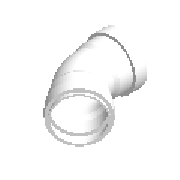
# Autodesk Inventor part: ISO 3633 45 Deg Bend with Only Sockets for Elastomeric Sealing Ring Joints DN160
Saved by Autodesk Inventor 2023.1 (Build 271208000, 208)
## iProperties
Created: 2022-02-04
Part Number: ISO 3633 45 Deg Bend with Only Sockets for Elastomeric Sealing Ring Joints DN160
Material: PVC, Unplasticized
Description: Unplasticized poly(vinylchloride) (PVC-U) - Bend with Only Sockets for Elastomeric Sealing Ring Joints
Document SubType Name: Modeling
Standard: ISO 3633
Designer: user
Standard Revision: Second edition 2002-09-01
Standards Organization: ISO
Language: en-US
Size Designation: DN160
Categories: <MemberInstance><Categories><Category DisplayName="Tube &amp; Pipe" InternalName="4347fa0f-2144-441d-94cd-e3e15c92b736" Mnemonic="TUBEANDPIPE"><CategoryParameter DisplayName="Number of Connections" InternalName="04e9c83a-9e20-4a98-a7e1-e8abe87a2846" Mnemonic="NUM_CONNECTIONS"/><CategoryParameter DisplayName="Angles" InternalName="0e0e4fa4-3bd3-4656-a22e-4e07c8c476f8" Mnemonic="ANGLES"><CategoryParameter DisplayName="Angle" InternalName="9188ad83-1b16-48b4-8b0a-76ce729dafa7" Mnemonic="ANGLE"/></CategoryParameter><CategoryParameter DisplayName="SKey" InternalName="3da84699-049a-4bc2-a65a-6696b77c242f" Mnemonic="SKEY"/><CategoryParameter DisplayName="ISOGEN Description" InternalName="7aa3ba45-b821-4467-8584-f9e6f15f2a7d" Mnemonic="ISOGENDESC"/><CategoryParameter DisplayName="ITEM-CODE" InternalName="99cc3b15-24d9-4d38-aac7-792cfbc57acf" Mnemonic="ITEMCODE"/><CategoryParameter DisplayName="NameOfComponent" InternalName="9c74ad13-48a1-45fe-b0f7-5447561f444a" Mnemonic="NAMEOFCOMPONENT"/><CategoryParameter DisplayName="InLineGroups" InternalName="d60be647-bc43-4c18-a13f-9fe4115f8e64" Mnemonic="INLINEGROUPS"/><Category DisplayName="Fittings" InternalName="ed6b26c4-72b8-4f31-9b63-f85ae8f932e4" Mnemonic="FITTINGS"><CategoryParameter DisplayName="Connections" InternalName="dbd721e8-e885-4eea-9011-b5acfd9f61de" Mnemonic="FIT_CONNECTIONS"><CategoryParameter DisplayName="Min Mating Pipe Size" InternalName="11f51b32-3e37-4310-abf7-f1318a1fd129" Mnemonic="MNMPS"/><CategoryParameter DisplayName="MaxEngagement" InternalName="34fdf028-8797-436e-ba07-ca3dee15bd9b" Mnemonic="MAXENGAGEMENT"/><CategoryParameter DisplayName="NominalSize" InternalName="3f94edc7-e459-48db-8f02-8eebf8cffccd" Mnemonic="NS"/><CategoryParameter DisplayName="DisplayName" InternalName="50f521dd-e050-43f7-9895-6b30ea7ed42e" Mnemonic="DISPLAYNAME"/><CategoryParameter DisplayName="Cut Mating Pipe" InternalName="53a63a6e-53d8-4ca9-8880-037731d1cceb" Mnemonic="CMP"/><CategoryParameter DisplayName="Gender Neutral" InternalName="628bd5f1-acad-44e2-9d91-af996ab74fc2" Mnemonic="NEUTRAL"/><CategoryParameter DisplayName="MinEngagement [% of MaxEngagement]" InternalName="7ec1bde5-73f0-45b1-98d8-365a6c67f8ad" Mnemonic="MINENGAGEMENT"/><CategoryParameter DisplayName="Fixed" InternalName="9142902a-6a8a-446d-9eb8-4b7ce7d245ef" Mnemonic="FIXED"/><CategoryParameter DisplayName="Female" InternalName="b366bcb5-a500-4bad-84bb-22f956216d69" Mnemonic="FEMALE"/><CategoryParameter DisplayName="FlipDirection" InternalName="d55dedc0-f14a-4283-86b4-a4eeb253c8aa" Mnemonic="FLIPDIRECTION"/><CategoryParameter DisplayName="ScheduleNumber" InternalName="d6161c62-eb59-4495-a086-874847c10866" Mnemonic="SN"/><CategoryParameter DisplayName="EndTreatment" InternalName="d7f11516-3374-45ca-b1c7-4b2d63244ae2" Mnemonic="ENDTREATMENT"/><CategoryParameter DisplayName="Max Mating Pipe Size" InternalName="e73ef66b-c04b-45ac-9b32-f712653e25ee" Mnemonic="MXMPS"/></CategoryParameter><CategoryParameter DisplayName="Connections" InternalName="dbd721e8-e885-4eea-9011-b5acfd9f61de" Mnemonic="FIT_CONNECTIONS"><CategoryParameter DisplayName="Min Mating Pipe Size" InternalName="11f51b32-3e37-4310-abf7-f1318a1fd129" Mnemonic="MNMPS"/><CategoryParameter DisplayName="MaxEngagement" InternalName="34fdf028-8797-436e-ba07-ca3dee15bd9b" Mnemonic="MAXENGAGEMENT"/><CategoryParameter DisplayName="NominalSize" InternalName="3f94edc7-e459-48db-8f02-8eebf8cffccd" Mnemonic="NS"/><CategoryParameter DisplayName="DisplayName" InternalName="50f521dd-e050-43f7-9895-6b30ea7ed42e" Mnemonic="DISPLAYNAME"/><CategoryParameter DisplayName="Cut Mating Pipe" InternalName="53a63a6e-53d8-4ca9-8880-037731d1cceb" Mnemonic="CMP"/><CategoryParameter DisplayName="Gender Neutral" InternalName="628bd5f1-acad-44e2-9d91-af996ab74fc2" Mnemonic="NEUTRAL"/><CategoryParameter DisplayName="MinEngagement [% of MaxEngagement]" InternalName="7ec1bde5-73f0-45b1-98d8-365a6c67f8ad" Mnemonic="MINENGAGEMENT"/><CategoryParameter DisplayName="Fixed" InternalName="9142902a-6a8a-446d-9eb8-4b7ce7d245ef" Mnemonic="FIXED"/><CategoryParameter DisplayName="Female" InternalName="b366bcb5-a500-4bad-84bb-22f956216d69" Mnemonic="FEMALE"/><CategoryParameter DisplayName="FlipDirection" InternalName="d55dedc0-f14a-4283-86b4-a4eeb253c8aa" Mnemonic="FLIPDIRECTION"/><CategoryParameter DisplayName="ScheduleNumber" InternalName="d6161c62-eb59-4495-a086-874847c10866" Mnemonic="SN"/><CategoryParameter DisplayName="EndTreatment" InternalName="d7f11516-3374-45ca-b1c7-4b2d63244ae2" Mnemonic="ENDTREATMENT"/><CategoryParameter DisplayName="Max Mating Pipe Size" InternalName="e73ef66b-c04b-45ac-9b32-f712653e25ee" Mnemonic="MXMPS"/></CategoryParameter><Category DisplayName="Elbows" InternalName="d634b27c-b107-44eb-a6d6-89e046173c17" Mnemonic="Elbow"/></Category></Category><Category DisplayName="DataType" InternalName="23b78d0f-2648-40c6-8793-ca6db495c9e8" Mnemonic="DATATYPE"><CategoryParameter DisplayName="DisplayName" InternalName="05415f3d-3907-474b-a020-eb9d644f4cf3" Mnemonic="DISPLAYNAME"/><CategoryParameter DisplayName="Standard" InternalName="0c0a119c-1e12-4c84-803f-101930972f5e" Mnemonic="STANDARD"/><CategoryParameter DisplayName="Description" InternalName="13903e3d-64b1-4950-80da-f627842ea37f" Mnemonic="DESCRIPTION"/><CategoryParameter DisplayName="Designation" InternalName="2675968c-4ce5-49e0-a4f5-552d29089031" Mnemonic="DESIGNATION"/><CategoryParameter DisplayName="Default Row" InternalName="2af9ec52-faaa-4026-b378-f9fa4afca842" Mnemonic="DEFAULTROW"/><CategoryParameter DisplayName="Folder Name" InternalName="3f06958e-8713-4116-9be7-ed6184ecc97b" Mnemonic="FOLDERNAME"/><CategoryParameter DisplayName="Revision Guid" InternalName="45a75005-10b1-4dfc-8d6d-dfe629f0b93c" Mnemonic="REVISIONGUID"/><CategoryParameter DisplayName="FileName" InternalName="8b46a4cc-9585-4fed-90c3-899f57e09a73" Mnemonic="FILENAME"/><CategoryParameter DisplayName="StdsOrg" InternalName="8f5914e1-4693-403f-8ab5-d37768198c9d" Mnemonic="STDSORG"/><CategoryParameter DisplayName="Family Version" InternalName="914462f6-6e19-4b14-ba84-155b9680b1d0" Mnemonic="FAMILYREVISION"/><CategoryParameter DisplayName="Standard Revision" InternalName="91d5a463-65c2-4fde-b823-3b7fea5e8e17" Mnemonic="STANDARDREVISION"/><CategoryParameter DisplayName="Member Revision" InternalName="a65d44b9-392f-4f4f-857b-e4b3d54996fe" Mnemonic="MEMBERREVISION"/><CategoryParameter DisplayName="ClipFormat" InternalName="bc51e27b-3422-4e78-93ef-cec197ddf230" Mnemonic="CLIPFORMAT"/><CategoryParameter DisplayName="Manufacturer" InternalName="cd6c7a72-a28a-4e50-99a9-2c7f4e13e5ad" Mnemonic="MANUFACTURER"/><CategoryParameter DisplayName="InternalName" InternalName="cf1d0246-76d9-4b4a-8305-fa0409afb5c1" Mnemonic="INTERNALNAME"/><CategoryParameter DisplayName="IsMetric" InternalName="e2385c5b-1ea4-4823-96a8-8de651266ec3" Mnemonic="ISMETRIC"/><Category DisplayName="Part" InternalName="c0e0b642-3bcb-4cc8-9e80-f96d35c4afa4" Mnemonic="PART"><CategoryParameter DisplayName="Part Number" InternalName="016b6077-bfbe-49bd-92c9-d8d59c39c941" Mnemonic="PARTNUMBER"/><CategoryParameter DisplayName="Stock Number" InternalName="4dba7c1c-e26c-444e-836c-b08b433409a8" Mnemonic="STOCKNUMBER"/><CategoryParameter DisplayName="Material Key" InternalName="5c9a8adb-dd2b-4535-b97f-0a94a95fe41f" Mnemonic="MATERIALKEY"/><CategoryParameter DisplayName="Material" InternalName="818a152a-d3c3-49ca-80ee-df7d91421b8e" Mnemonic="MATERIAL"/></Category></Category><Category DisplayName="LegacyMap" InternalName="dfeab48a-acc2-4514-a11c-1b8dc28c3d5f" Mnemonic="LEGACYMAP"><CategoryParameter DisplayName="CatalogID" InternalName="0da51c36-8fd3-4028-86cc-0c9c9e96136a" Mnemonic="CATALOGID"/><CategoryParameter DisplayName="FamilyID" InternalName="1c0b589c-8bbe-4e1e-80cf-07c0de42ac2a" Mnemonic="FAMILYID"/><CategoryParameter DisplayName="MemberID" InternalName="a368ea03-db8a-4d6e-962b-2aa46306b8f5" Mnemonic="MEMBERID"/></Category></Categories><FamilyTemplate Id="ISO 3633 45 Deg Bend with Only Sockets for Elastomeric Sealing Ring Joints"><FamilyTemplateParameters><FamilyTemplateParameter ObjectType="kUserParameterObject" ValueType="xs:double" Id="1" ObjectReferenceKey="z"/><FamilyTemplateParameter ObjectType="kUserParameterObject" ValueType="xs:double" Id="2" ObjectReferenceKey="De"/><FamilyTemplateParameter ObjectType="kUserParameterObject" ValueType="xs:double" Id="3" ObjectReferenceKey="e"/><FamilyTemplateParameter ObjectType="kUserParameterObject" ValueType="xs:double" Id="4" ObjectReferenceKey="Ds"/><FamilyTemplateParameter ObjectType="kUserParameterObject" ValueType="xs:double" Id="5" ObjectReferenceKey="C1"/><FamilyTemplateParameter ObjectType="kUserParameterObject" ValueType="xs:double" Id="6" ObjectReferenceKey="A"/><FamilyTemplateParameter ObjectType="kUserParameterObject" ValueType="xs:string" Id="116" ObjectReferenceKey="Size_Designation"/><FamilyTemplateParameter ObjectType="kPropertyObject" ValueType="xs:string" Id="100" ObjectReferenceKey="{32853F0F-3444-11d1-9E93-0060B03C1CA6}" SubObjectId="52"/><FamilyTemplateParameter ObjectType="kPropertyObject" ValueType="xs:string" Id="105" ObjectReferenceKey="{32853F0F-3444-11d1-9E93-0060B03C1CA6}" SubObjectId="5"/><FamilyTemplateParameter ObjectType="kPartComponentDefinitionObject" ValueType="xs:string" Id="110" SubObjectId="Material"/></FamilyTemplateParameters></FamilyTemplate><CategoryParameterMap><ParamToTemplateMap><ParamToTemplate CategoryParameter="//CategoryParameter[@InternalName='d60be647-bc43-4c18-a13f-9fe4115f8e64']" ConstantValue="0"/><ParamToTemplate CategoryParameter="//CategoryParameter[@InternalName='04e9c83a-9e20-4a98-a7e1-e8abe87a2846']" ConstantValue="2"/><ParamToTemplate CategoryParameter="//CategoryParameter[@InternalName='0e0e4fa4-3bd3-4656-a22e-4e07c8c476f8']" ConstantValue=""/><ParamToTemplate CategoryParameter="//CategoryParameter[@InternalName='0e0e4fa4-3bd3-4656-a22e-4e07c8c476f8'][1]/CategoryParameter[@InternalName='9188ad83-1b16-48b4-8b0a-76ce729dafa7']" ConstantValue="2.35619449019234"/><ParamToTemplate CategoryParameter="//CategoryParameter[@InternalName='9c74ad13-48a1-45fe-b0f7-5447561f444a']" ConstantValue="ELBOW"/><ParamToTemplate CategoryParameter="//CategoryParameter[@InternalName='3da84699-049a-4bc2-a65a-6696b77c242f']" ConstantValue="ELPF"/><ParamToTemplate CategoryParameter="//CategoryParameter[@InternalName='dbd721e8-e885-4eea-9011-b5acfd9f61de'][1]/CategoryParameter[@InternalName='d55dedc0-f14a-4283-86b4-a4eeb253c8aa']" ConstantValue="true"/><ParamToTemplate CategoryParameter="//CategoryParameter[@InternalName='dbd721e8-e885-4eea-9011-b5acfd9f61de'][1]/CategoryParameter[@InternalName='50f521dd-e050-43f7-9895-6b30ea7ed42e']" ConstantValue="Connection1"/><ParamToTemplate CategoryParameter="//CategoryParameter[@InternalName='dbd721e8-e885-4eea-9011-b5acfd9f61de'][1]/CategoryParameter[@InternalName='b366bcb5-a500-4bad-84bb-22f956216d69']" ConstantValue="true"/><ParamToTemplate CategoryParameter="//CategoryParameter[@InternalName='dbd721e8-e885-4eea-9011-b5acfd9f61de'][1]/CategoryParameter[@InternalName='d7f11516-3374-45ca-b1c7-4b2d63244ae2']" ConstantValue="Jointed"/><ParamToTemplate CategoryParameter="//CategoryParameter[@InternalName='dbd721e8-e885-4eea-9011-b5acfd9f61de'][1]/CategoryParameter[@InternalName='9142902a-6a8a-446d-9eb8-4b7ce7d245ef']" ConstantValue="false"/><ParamToTemplate CategoryParameter="//CategoryParameter[@InternalName='dbd721e8-e885-4eea-9011-b5acfd9f61de'][1]/CategoryParameter[@InternalName='34fdf028-8797-436e-ba07-ca3dee15bd9b']" ConstantValue="0"/><ParamToTemplate CategoryParameter="//CategoryParameter[@InternalName='dbd721e8-e885-4eea-9011-b5acfd9f61de'][1]/CategoryParameter[@InternalName='7ec1bde5-73f0-45b1-98d8-365a6c67f8ad']" ConstantValue="20"/><ParamToTemplate CategoryParameter="//CategoryParameter[@InternalName='dbd721e8-e885-4eea-9011-b5acfd9f61de'][2]/CategoryParameter[@InternalName='d55dedc0-f14a-4283-86b4-a4eeb253c8aa']" ConstantValue="false"/><ParamToTemplate CategoryParameter="//CategoryParameter[@InternalName='dbd721e8-e885-4eea-9011-b5acfd9f61de'][2]/CategoryParameter[@InternalName='50f521dd-e050-43f7-9895-6b30ea7ed42e']" ConstantValue="Connection2"/><ParamToTemplate CategoryParameter="//CategoryParameter[@InternalName='dbd721e8-e885-4eea-9011-b5acfd9f61de'][2]/CategoryParameter[@InternalName='b366bcb5-a500-4bad-84bb-22f956216d69']" ConstantValue="true"/><ParamToTemplate CategoryParameter="//CategoryParameter[@InternalName='dbd721e8-e885-4eea-9011-b5acfd9f61de'][2]/CategoryParameter[@InternalName='d7f11516-3374-45ca-b1c7-4b2d63244ae2']" ConstantValue="Jointed"/><ParamToTemplate CategoryParameter="//CategoryParameter[@InternalName='dbd721e8-e885-4eea-9011-b5acfd9f61de'][2]/CategoryParameter[@InternalName='9142902a-6a8a-446d-9eb8-4b7ce7d245ef']" ConstantValue="false"/><ParamToTemplate CategoryParameter="//CategoryParameter[@InternalName='dbd721e8-e885-4eea-9011-b5acfd9f61de'][2]/CategoryParameter[@InternalName='34fdf028-8797-436e-ba07-ca3dee15bd9b']" ConstantValue="0"/><ParamToTemplate CategoryParameter="//CategoryParameter[@InternalName='dbd721e8-e885-4eea-9011-b5acfd9f61de'][2]/CategoryParameter[@InternalName='7ec1bde5-73f0-45b1-98d8-365a6c67f8ad']" ConstantValue="20"/><ParamToTemplate CategoryParameter="//CategoryParameter[@InternalName='05415f3d-3907-474b-a020-eb9d644f4cf3']" ConstantValue="ISO 3633 45 Deg Bend with Only Sockets for Elastomeric Sealing Ring Joints"/><ParamToTemplate CategoryParameter="//CategoryParameter[@InternalName='cf1d0246-76d9-4b4a-8305-fa0409afb5c1']" ConstantValue="421a8b99-1721-409a-bc3b-c00889561754"/><ParamToTemplate CategoryParameter="//CategoryParameter[@InternalName='3f06958e-8713-4116-9be7-ed6184ecc97b']" ConstantValue="ISO 3633 45 (01)"/><ParamToTemplate CategoryParameter="//CategoryParameter[@InternalName='914462f6-6e19-4b14-ba84-155b9680b1d0']" ConstantValue="10"/><ParamToTemplate CategoryParameter="//CategoryParameter[@InternalName='13903e3d-64b1-4950-80da-f627842ea37f']" ConstantValue="Unplasticized poly(vinylchloride) (PVC-U) - Bend with Only Sockets for Elastomeric Sealing Ring Joints"/><ParamToTemplate CategoryParameter="//CategoryParameter[@InternalName='8f5914e1-4693-403f-8ab5-d37768198c9d']" ConstantValue="ISO"/><ParamToTemplate CategoryParameter="//CategoryParameter[@InternalName='0c0a119c-1e12-4c84-803f-101930972f5e']" ConstantValue="ISO 3633"/><ParamToTemplate CategoryParameter="//CategoryParameter[@InternalName='cd6c7a72-a28a-4e50-99a9-2c7f4e13e5ad']" TemplateParameter="104"/><ParamToTemplate CategoryParameter="//CategoryParameter[@InternalName='91d5a463-65c2-4fde-b823-3b7fea5e8e17']" ConstantValue="Second edition 2002-09-01"/><ParamToTemplate CategoryParameter="//CategoryParameter[@InternalName='bc51e27b-3422-4e78-93ef-cec197ddf230']" ConstantValue="CF_INVENTOR.STDPARTS"/><ParamToTemplate CategoryParameter="//CategoryParameter[@InternalName='e2385c5b-1ea4-4823-96a8-8de651266ec3']" ConstantValue="true"/><ParamToTemplate CategoryParameter="//CategoryParameter[@InternalName='45a75005-10b1-4dfc-8d6d-dfe629f0b93c']" ConstantValue="7111df97-f606-461c-b42e-48126bad22a5"/><ParamToTemplate CategoryParameter="//CategoryParameter[@InternalName='2af9ec52-faaa-4026-b378-f9fa4afca842']" ConstantValue="3"/><ParamToTemplate CategoryParameter="//CategoryParameter[@InternalName='0da51c36-8fd3-4028-86cc-0c9c9e96136a']" ConstantValue="1B06E4C7-776A-41B3-A0ED-A3EE7199E845"/><ParamToTemplate CategoryParameter="//CategoryParameter[@InternalName='1c0b589c-8bbe-4e1e-80cf-07c0de42ac2a']" ConstantValue="421a8b99-1721-409a-bc3b-c00889561754"/><ParamToTemplate CategoryParameter="//CategoryParameter[@InternalName='99cc3b15-24d9-4d38-aac7-792cfbc57acf']" ConstantValue=""/><ParamToTemplate CategoryParameter="//CategoryParameter[@InternalName='7aa3ba45-b821-4467-8584-f9e6f15f2a7d']" ConstantValue=""/><ParamToTemplate CategoryParameter="//CategoryParameter[@InternalName='dbd721e8-e885-4eea-9011-b5acfd9f61de'][1]/CategoryParameter[@InternalName='3f94edc7-e459-48db-8f02-8eebf8cffccd']" ConstantValue="M160"/><ParamToTemplate CategoryParameter="//CategoryParameter[@InternalName='dbd721e8-e885-4eea-9011-b5acfd9f61de'][2]/CategoryParameter[@InternalName='3f94edc7-e459-48db-8f02-8eebf8cffccd']" ConstantValue="M160"/><ParamToTemplate CategoryParameter="//CategoryParameter[@InternalName='8b46a4cc-9585-4fed-90c3-899f57e09a73']" ConstantValue="ISO 3633 45 Deg Bend with Only Sockets for Elastomeric Sealing Ring Joints DN160"/><ParamToTemplate CategoryParameter="//CategoryParameter[@InternalName='a65d44b9-392f-4f4f-857b-e4b3d54996fe']" ConstantValue="1E3F9FC1-313A-4622-90BA-1049764EA002"/><ParamToTemplate CategoryParameter="//CategoryParameter[@InternalName='a368ea03-db8a-4d6e-962b-2aa46306b8f5']" ConstantValue="2B7A464F-B7A7-421C-8A8B-63B1B6CA7584"/><ParamToTemplate CategoryParameter="//CategoryParameter[@InternalName='2675968c-4ce5-49e0-a4f5-552d29089031']" TemplateParameter="100"/><ParamToTemplate CategoryParameter="//CategoryParameter[@InternalName='818a152a-d3c3-49ca-80ee-df7d91421b8e']" TemplateParameter="110"/><ParamToTemplate CategoryParameter="//CategoryParameter[@InternalName='016b6077-bfbe-49bd-92c9-d8d59c39c941']" TemplateParameter="105"/></ParamToTemplateMap></CategoryParameterMap></MemberInstance>
Density: 1.29 g/cm^3
Appearance: Smooth - White
IsCustomPart: 0
NAME: PIPING: ISO 3633 45 Deg Bend with Only Sockets for Elastomeric Sealing Ring Joints
DATA: <meta><inlinegroups number="0" deflen="0"></inlinegroups><connections number="2"></connections><angles><a>2.35619449019234</a></angles></meta>
Author: user
Autodesk Inventor part; units mm, degrees
ref_plane "YZ Plane" through (0, 0, 0) normal (1, 0, 0) x (0, 1, 0)
ref_plane "XZ Plane" through (0, 0, 0) normal (0, 1, 0) x (-1, 0, 0)
ref_plane "XY Plane" through (0, 0, 0) normal (0, 0, 1) x (1, 0, 0)
sketch "Sketch1" plane through (0, 0, 0) normal (0, 1, 0) x (-1, 0, 0)
  line L0 (0, 0) -> (0, 81.1234)
  line L1 (76.8, 81.1234) -> (80, 81.1234)
  line L2 (0, 81.1234) -> (76.8, 81.1234) construction
  line L3 (80, 81.1234) -> (83.13, 74.6607)
  line L4 (83.13, 34.4) -> (87.45, 34.4)
  line L5 (87.45, 34.4) -> (87.45, 8.8)
  line L6 (87.45, 8.8) -> (82.65, 8.8)
  line L7 (82.65, 8.8) -> (82.65, 0)
  line L8 (82.65, 0) -> (80.25, 0)
  line L9 (80.25, 0) -> (80.25, 11.2)
  line L10 (80.25, 11.2) -> (85.05, 11.2)
  line L11 (85.05, 11.2) -> (85.05, 32)
  line L12 (85.05, 32) -> (80.25, 32)
  line L13 (80.25, 32) -> (80.25, 74)
  line L14 (80.25, 74) -> (76.8, 81.1234)
  line L15 (80.25, 0) -> (0, 0) construction
  line L16 (83.13, 74.6607) -> (83.13, 34.4)
  line L17 (0, 81.1234) -> (0, 123.1234) construction
  line L18 (0, 123.1234) -> (-29.6985, 152.8218) construction
  line L19 (-29.6985, 152.8218) -> (-87.0614, 210.1847) construction
  line L20 (-87.0614, 210.1847) -> (-30.316, 266.93) construction
  line L21 (-30.316, 266.93) -> (-28.619, 268.6271)
  line L22 (-28.619, 268.6271) -> (-22.3964, 262.4046)
  line L23 (-22.3964, 262.4046) -> (-19.0023, 265.7987)
  line L24 (-19.0023, 265.7987) -> (-0.9004, 247.6967)
  line L25 (-0.9004, 247.6967) -> (-3.9551, 244.642)
  line L26 (-3.9551, 244.642) -> (24.5135, 216.1734)
  line L27 (24.5135, 216.1734) -> (26.8701, 209.3904)
  line L28 (26.8701, 209.3904) -> (24.6073, 207.1276)
  line L29 (24.6073, 207.1276) -> (22.0099, 214.6041)
  line L30 (22.0099, 214.6041) -> (-7.6886, 244.3026)
  line L31 (-7.6886, 244.3026) -> (-4.2945, 247.6967)
  line L32 (-4.2945, 247.6967) -> (-19.0023, 262.4046)
  line L33 (-19.0023, 262.4046) -> (-22.3964, 259.0104)
  line L34 (-22.3964, 259.0104) -> (-30.316, 266.93)
  line L35 (24.6073, 207.1276) -> (-29.6985, 152.8218) construction
  line L36 (80.25, 74) -> (0, 74) construction
  line L37 (22.0099, 214.6041) -> (-34.7355, 157.8588) construction
  dimension "d0" = 2.4
  dimension "d1" = 2.4
  dimension "d2" = 2.4
  dimension "d4" = 2.88
  dimension "d5" = 2.4
  dimension "d6" = 7.2
  dimension "d7" = 160.5
  dimension "d8" = 32
  dimension "d9" = 42
  dimension "d11" = 11.2
  dimension "d12" = 160
  dimension "d13" = 3.2
  dimension "d14" = 2.88
  dimension "d18" = 160.5
  dimension "d19" = 2.4
  dimension "d20" = 2.4
  dimension "d21" = 2.4
  dimension "d22" = 2.4
  dimension "d23" = 4.8
  dimension "d24" = 2.88
  dimension "d25" = 3.2
  dimension "d26" = 160
  dimension "d27" = 11.2
  dimension "d28" = 32
  dimension "d29" = 42
  dimension "d30" = 45
  dimension "d31" = 42
  dimension "d32" = 42
  dimension "d33" = 2.88
  constraints: 76 end point, 23 perpendicular, 7 collinear, 6 parallel, 2 point on line, 1 horizontal, 1 vertical
  measures "d0" distance between parallel lines of L9 L7
  measures "d1" distance between parallel lines of L5 L11
  measures "d2" distance between parallel lines of L4 L12
  measures "d4" distance between parallel lines of L3 L14
  measures "d5" distance between parallel lines of L10 L6
  measures "d6" distance between parallel lines of L9 L5
  measures "d7" diameter of L9 L0
  measures "d8" distance between parallel lines of L8 L12
  measures "d9" distance from line of L12 L13.end
  measures "d11" distance of L8.end L9.end
  measures "d12" diameter of L1.end L0
  measures "d13" distance of L1.start L1.end
  measures "d14" distance between parallel lines of L16 L13
  measures "d18" diameter of L34 L19
  measures "d19" distance between parallel lines of L22 L34
  measures "d20" distance between parallel lines of L33 L23
  measures "d21" distance between parallel lines of L32 L24
  measures "d22" distance between parallel lines of L31 L25
  measures "d23" distance between parallel lines of L22 L24
  measures "d24" distance between parallel lines of L30 L26
  measures "d25" distance of L27.end L28.end
  measures "d26" diameter of L27.end L19
  measures "d27" distance of L33.end L20.end
  measures "d28" distance between parallel lines of L31 L21
  measures "d29" distance from line of L29.end L31
  measures "d30" angle of L17 L18
  measures "d31" distance of L0.end L17.end
  measures "d32" distance of L17.end L18.end
  measures "d33" distance between parallel lines of L29 L27
revolve "Revolution1" add sketch "Sketch1" angle 360 about axis through (0, 0, 0) along (0, 0, 1) contours L1 L3 L16 L4 L5 L6 L7 L8 L9 L10 L11 L12 L13 L14
sketch "Sketch2" plane through (0, 0, 81.1234) normal (0, 0, 1) x (1, 0, 0)
  circle A0 centre (0, 0) radius 80 projected
  circle A1 centre (0, 0) radius 80
  circle A2 centre (0, 0) radius 76.8
  circle A3 centre (0, 0) radius 76.8 projected
  constraints: 4 concentric, 2 centre point, 2 coincident
sketch "Sketch3" plane through (0, 0, 0) normal (0, 1, 0) x (-1, 0, 0)
  line L0 (-80, 81.1234) -> (80, 81.1234) projected
  line L1 (0, 81.1234) -> (0, 123.1234) construction
  line L2 (0, 123.1234) -> (-29.6985, 152.8218) construction
  arc A0 (0, 81.1234) -> (-29.6985, 152.8218) centre (-101.397, 81.1234) ccw
  dimension "d15" = 45
  dimension "d16" = 42
  dimension "d17" = 42
  constraints: 4 end point, 2 point on circle, 1 centre point, 1 midpoint, 1 perpendicular, 1 tangent
  measures "d15" angle of L1 L2
  measures "d16" distance of L1.start L1.end
  measures "d17" distance of L1.end L2.end
sweep "Sweep1" add profiles "Sketch2" path "Sketch3" path curves A0
revolve "Revolution2" add sketch "Sketch1" angle 360 about axis through (29.6985, 0, 152.8218) along (0.7071068, 0, 0.7071068) contours L21 L22 L23 L24 L25 L26 L27 L28 L29 L30 L31 L32 L33 L34
equation "\"d0\" = e3"
equation "\"d1\" = e3"
equation "\"d2\" = e3"
equation "\"d4\" = e2"
equation "\"d5\" = e3"
equation "\"d6\" = 3 * e3"
equation "\"d7\" = Ds"
equation "\"d8\" = C1"
equation "\"d9\" = A"
equation "\"d11\" = 0.35 * C1"
equation "\"d12\" = De"
equation "\"d13\" = e"
equation "\"d14\" = e2"
equation "\"d18\" = Ds"
equation "\"d19\" = e3"
equation "\"d20\" = e3"
equation "\"d21\" = e3"
equation "\"d22\" = e3"
equation "\"d23\" = 2 * e3"
equation "\"d24\" = e2"
equation "\"d25\" = e"
equation "\"d26\" = De"
equation "\"d27\" = 0.35 * C1"
equation "\"d28\" = C1"
equation "\"d29\" = A"
equation "\"d31\" = z"
equation "\"d32\" = z"
equation "\"d33\" = e2"
equation "\"d16\" = z"
equation "\"d17\" = z"
equation "\"z\" = 42"
equation "\"De\" = 160"
equation "\"e\" = 3.2"
equation "\"Ds\" = 160.5"
equation "\"e2\" = 0.9 * e"
equation "\"C1\" = 32"
equation "\"e3\" = 0.75 * e"
equation "\"A\" = 42"
equation "\"Size_Designation\" = 1.2345"
body "Solid1"
